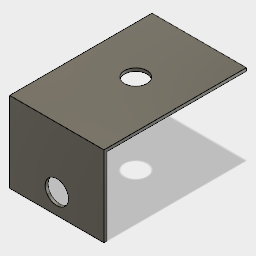
top shell v2 v2 (Autodesk Fusion 360 design; units mm, degrees)
Autodesk Fusion 360 part; units mm, degrees
sketch "Sketch1" plane through (0, 0, 0) normal (0, 0, 1) x (1, 0, 0)
  line L0 (15.25, -12.5) -> (-15.25, -12.5)
  line L1 (-15.25, -12.5) -> (-15.25, 12.5)
  line L2 (-15.25, 12.5) -> (15.25, 12.5)
  line L3 (15.25, 12.5) -> (15.25, -12.5)
  line L4 (15.25, -12.5) -> (-15.25, 12.5) construction
  line L5 (-15.25, -12.5) -> (15.25, 12.5) construction
  dimension "d1" = 30.5
  dimension "d2" = 25
  measures "d1" distance of L1.end L2.end
  measures "d2" distance of L0.end L1.end
extrude "Extrude1" add sketch "Sketch1" along normal blind 1
sketch "Sketch2" plane through (0, 12.5, 0) normal (0, 1, 0) x (-1, 0, 0)
  line L0 (-15.25, 0) -> (15.25, 0)
  line L1 (15.25, 0) -> (15.25, 1)
  line L2 (15.25, 1) -> (-15.25, 1)
  line L3 (-15.25, 1) -> (-15.25, 0)
  line L4 (15.25, 1) -> (-15.25, 1)
  line L5 (-15.25, 1) -> (-15.25, -45)
  line L6 (-15.25, -45) -> (15.25, -45)
  line L7 (15.25, -45) -> (15.25, 1)
  dimension "d5" = 46
  dimension "d6" = 30.5
  measures "d5" distance of L1.end L6.end
  measures "d6" distance of L1.end L2.end
extrude "Extrude2" add sketch "Sketch2" along normal blind 1
sketch "Sketch3" plane through (0, 0, 1) normal (0, 0, 1) x (1, 0, 0)
  line L0 (-15.25, 13.5) -> (-15.25, -12.5)
  line L1 (-15.25, -12.5) -> (15.25, -12.5)
  line L2 (15.25, -12.5) -> (15.25, 13.5)
  line L3 (15.25, 13.5) -> (-15.25, 13.5)
  line L4 (0, -12.5) -> (0, -5.95)
  circle A0 centre (0, -5.95) radius 3.75
  dimension "d9" = 6.55
  dimension "d10" = 7.5
  measures "d9" distance of L4.start L4.end
  measures "d10" diameter of A0
extrude "Extrude3" cut sketch "Sketch3" against normal blind 46 contours A0
sketch "Sketch4" plane through (0, 13.5, 0) normal (0, 1, 0) x (-1, 0, 0)
  line L0 (15.25, -45) -> (15.25, 1)
  line L1 (15.25, 1) -> (-15.25, 1)
  line L2 (-15.25, 1) -> (-15.25, -45)
  line L3 (-15.25, -45) -> (15.25, -45)
  line L4 (0, 1) -> (0, -24.5)
  circle A0 centre (0, -24.5) radius 3.625
  dimension "d13" = 25.5
  dimension "d14" = 7.25
  measures "d13" distance of L4.start L4.end
  measures "d14" diameter of A0
extrude "Extrude4" cut sketch "Sketch4" against normal blind 20 contours A0
equation "d9 = 2.8 mm + 3.75 mm"
